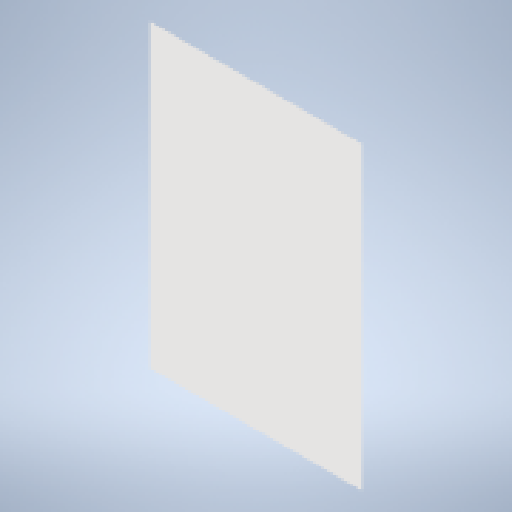
# Autodesk Inventor part: PaperA2
Saved by Autodesk Inventor 2023 (Build 270158000, 158)
## iProperties
Created: 2023-08-12
Part Number: PaperA2
Material: Paper
Document SubType Name: Modeling
Designer: Felix
Density: 0.93 g/cm^3
Appearance: Cardboard - Chipboard
Author: Felix
Autodesk Inventor part; units mm, degrees
ref_plane "YZ Plane" through (0, 0, 0) normal (1, 0, 0) x (0, 1, 0)
ref_plane "XZ Plane" through (0, 0, 0) normal (0, 1, 0) x (-1, 0, 0)
ref_plane "XY Plane" through (0, 0, 0) normal (0, 0, 1) x (1, 0, 0)
sketch "Sketch1" plane through (0, 0, 0) normal (0, 0, 1) x (1, 0, 0)
  line L0 (210, 297) -> (-210, 297)
  line L1 (-210, 297) -> (-210, -297)
  line L2 (-210, -297) -> (210, -297)
  line L3 (210, -297) -> (210, 297)
  line L4 (210, 297) -> (-210, -297) construction
  line L5 (-210, 297) -> (210, -297) construction
  point P0 (0, 0)
  dimension "d0" = 420
  dimension "d1" = 594
  constraints: 12 end point, 2 midpoint, 2 parallel, 1 horizontal, 1 perpendicular
  measures "d0" distance of L2.end L1.end
  measures "d1" distance of L1.end L0.end
extrude "Extrusion1" add sketch "Sketch1" along normal blind 0.1
body "Solid1"
